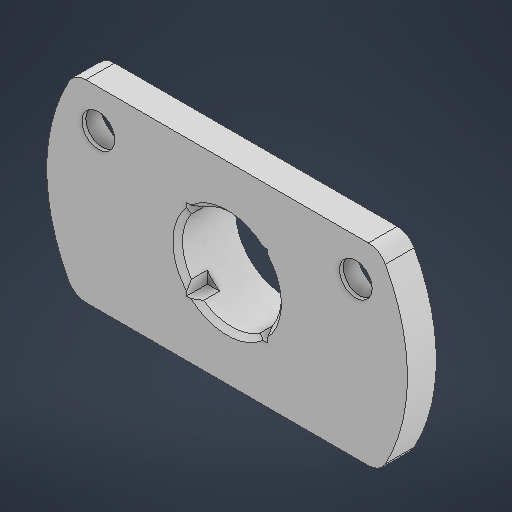
# Autodesk Inventor part: Držák-Cam+ir V2
Saved by Autodesk Inventor 2026 (Build 300175000, 175)
## iProperties
Created: 2025-06-20
Part Number: Držák-Cam+ir V2
Material: Všeobecné
Document SubType Name: Modeling
Designer: vadim
Density: 1 g/cm^3
Appearance: Výchozí
Author: vadim
Autodesk Inventor part; units mm, degrees
ref_plane "YZ Plane" through (0, 0, 0) normal (1, 0, 0) x (0, 1, 0)
ref_plane "XZ Plane" through (0, 0, 0) normal (0, 1, 0) x (-1, 0, 0)
ref_plane "XY Plane" through (0, 0, 0) normal (0, 0, 1) x (1, 0, 0)
sketch "Náčrt1" plane through (0, 0, 0) normal (0, 0, 1) x (1, 0, 0)
  circle A0 centre (0, 0) radius 5.125
  arc A1 (8.5, -16.6565) -> (-8.5, -16.6565) centre (0, 0) ccw
  line L0 (-13.35, 6.1) -> (13.35, 6.1)
  line L1 (0, 18.7) -> (0, -18.7)
  line L2 (8.5, -16.6565) -> (8.5, -22.2)
  line L3 (8.5, -22.2) -> (-8.5, -22.2)
  line L4 (-8.5, -22.2) -> (-8.5, -16.6565)
  line L5 (0, -18.7) -> (8.5, -22.2) construction
  line L6 (0, -18.7) -> (-8.5, -22.2) construction
  circle A2 centre (-13.35, 6.1) radius 1.7
  circle A3 centre (13.35, 6.1) radius 1.7
  line L7 (-12.1033, 10) -> (12.1033, 10)
  arc A4 (12.1033, 10) -> (-12.1033, 10) centre (0, 0) ccw
  line L8 (4.2, 4.2) -> (-4.2, 4.2)
  line L9 (-4.2, 4.2) -> (-4.2, -4.2)
  line L10 (-4.2, -4.2) -> (4.2, -4.2)
  line L11 (4.2, -4.2) -> (4.2, 4.2)
  line L12 (4.2, 4.2) -> (-4.2, -4.2) construction
  line L13 (-4.2, 4.2) -> (4.2, -4.2) construction
  line L14 (-3.55, -20.2) -> (3.55, -20.2)
  line L15 (3.55, -20.2) -> (3.55, -17.1)
  line L16 (3.55, -17.1) -> (-3.55, -17.1)
  line L17 (-3.55, -17.1) -> (-3.55, -20.2)
  line L18 (-3.55, -20.2) -> (3.55, -17.1) construction
  line L19 (3.55, -20.2) -> (-3.55, -17.1) construction
  circle A5 centre (0, 0) radius 5.575
  circle A6 centre (0, 0) radius 18.7
  circle A7 centre (-13.35, 6.1) radius 3
  circle A8 centre (13.35, 6.1) radius 3
  line L20 (-17.6407, 10) -> (18.7, 10)
  line L21 (0, 0) -> (-2.6642, 0) construction
  line L22 (-17.6407, -10) -> (18.7, -10)
  point P0 (-10.088, 6.1)
  point P1 (4.2, -2.9369)
  point P2 (2.9369, -4.2)
  point P3 (-2.9369, -4.2)
  point P4 (-4.2, -2.9369)
  point P5 (-4.2, 2.9369)
  point P6 (-2.9369, 4.2)
  point P7 (4.2, 2.9369)
  point P8 (2.9369, 4.2)
  point P9 (0, -18.65)
  point P10 (-8.5, -16.6565)
  point P11 (15.8016, -10)
  point P12 (15.8016, 10)
  point P13 (-15.8016, 10)
  point P14 (-15.8016, -10)
  dimension "d0" = 10.25
  dimension "d1" = 37.4
  dimension "d2" = 26.7
  dimension "d3" = 17
  dimension "d5" = 22.2
  dimension "d7" = 6.1
  dimension "d9" = 3.4
  dimension "d10" = 3.4
  dimension "d12" = 10
  dimension "d14" = 3
  dimension "d25" = 8.4
  dimension "d26" = 8.4
  dimension "d31" = 3.1
  dimension "d32" = 7.1
  dimension "d33" = 2
  dimension "d39" = 0.45
  dimension "d40" = 6
  dimension "d41" = 6
  constraints: 46 end point, 9 coincident, 8 centre point, 6 midpoint, 5 horizontal, 5 parallel, 5 point on circle, 3 perpendicular, 3 point on line, 3 symmetric about line, 1 vertical, 4 other
  measures "d0" diameter of A0
  measures "d1" diameter of A1
  measures "d2" distance of L0.start L0.end
  measures "d3" distance of L2.end L3.end
  measures "d5" distance from line of L3 point (0, 0)
  measures "d7" vertical distance of point (0, 0) L0.start
  measures "d9" diameter of A2
  measures "d10" diameter of A3
  measures "d12" distance from line of L7 A1.centre
  measures "d14" radial gap between concentric circles of A1 A4
  measures "d25" distance of L10.end L9.end
  measures "d26" distance of L9.end L8.end
  measures "d31" distance of L15.end L14.end
  measures "d32" distance of L15.end L16.end
  measures "d33" distance between parallel lines of L3 L14
  measures "d39" radial gap between concentric circles of A0 A5
  measures "d40" diameter of A7
  measures "d41" diameter of A8
extrude "Vysunutí1" add sketch "Náčrt1" along normal blind 0.4 contours A0 L11 A5 | A0 L8 A5 L11 | L11 A5 L10 A0 | A0 L1 A5 L8 | A5 L8 L11 | L11 L8 A5 L1 L7 L20 A1 L22 L10 | L10 A5 L1 A0 | L11 L10 A5 | A0 L8 A5 L1 | L1 A5 L10 A0 | A0 L9 A5 L8 | A5 L8 L9 L10 L1 L22 A1 L20 L7 | L10 A5 L9 A0 | A0 L9 A5 | A5 L9 L8 | L10 L9 A5 | A7 | A8
extrude "Vysunutí2" add sketch "Náčrt1" against normal blind 2.6 contours A0 L11 A5 | A0 L8 A5 L11 | L11 A5 L10 A0 | A0 L1 A5 L8 | A5 L8 L11 | L11 L8 A5 L1 L7 L20 A1 L22 L10 | L10 A5 L1 A0 | L11 L10 A5 | A0 L8 A5 L1 | L1 A5 L10 A0 | A0 L9 A5 L8 | A5 L8 L9 L10 L1 L22 A1 L20 L7 | L10 A5 L9 A0 | A0 L9 A5 | A5 L9 L8 | L10 L9 A5
chamfer "Zkosení1" distance 0.5 angle 45 1 edges at (-5.125, 0, 0.4)
extrude "Vysunutí3" cut sketch "Náčrt1" along normal blind 0.75 and the other way blind 1.75 contours A0 L8 A5 L11 | L11 A5 L10 A0 | A5 L8 L11 | L11 L10 A5 | A0 L9 A5 L8 | L10 A5 L9 A0 | A5 L9 L8 | L10 L9 A5
sketch "Náčrt2" plane through (0, 0, -2.6) normal (0, 0, -1) x (-1, 0, 0)
  circle A0 centre (0, 0) radius 5.125 projected
  circle A1 centre (0, 0) radius 5.7
  dimension "d35" = 11.4
  constraints: 1 centre point, 1 coincident
  measures "d35" diameter of A1
extrude "Vysunutí4" add sketch "Náčrt2" along normal blind 3
fillet "Zaoblení4" radius 0.5 1 edges at (5.7, 0, -2.6)
fillet "Zaoblení5" radius 2 4 edges at (15.8016, 10, -1.1) (-15.8016, 10, -1.1) (-15.8016, -10, -1.1) (15.8016, -10, -1.1)
